Autodesk Inventor part; units mm, degrees
(part 3 of 5)
  line L98 (0, 22) -> (0, -22) construction
  circle A131 centre (-90.3659, 45.1111) radius 1.6
  circle A132 centre (-45.1111, 90.3659) radius 1.6
  circle A133 centre (90.3659, -45.1111) radius 1.6
  circle A134 centre (45.1111, -90.3659) radius 1.6
  circle A135 centre (90.3659, 45.1111) radius 1.6
  circle A136 centre (45.1111, 90.3659) radius 1.6
  line L99 (41.3657, 27.2236) -> (27.2236, 41.3657) construction
  line L100 (34.2947, 34.2947) -> (55.1543, 55.1543) construction
  line L101 (46.669, 63.6396) -> (63.6396, 46.669) construction
  line L102 (0, 0) -> (0, -61.2072) construction
  circle A137 centre (0, -54) radius 1.6
  arc A138 (3.4868, -52.0398) -> (-3.4868, -52.0398) centre (0, -54) ccw
  line L103 (-0.6161, -51.9466) -> (-14.5119, -56.4463) construction
  line L104 (-5.1776, -53.4237) -> (-14.5119, -56.4463) construction
  line L105 (14.5119, -56.4463) -> (0.6161, -51.9466) construction
  line L106 (5.1776, -53.4237) -> (14.5119, -56.4463) construction
  arc A139 (0, -58) -> (3.8733, -53.0013) centre (0, -54) ccw construction
  arc A140 (-3.8733, -53.0013) -> (0, -58) centre (0, -54) ccw construction
  arc A141 (-5.1776, -53.4237) -> (-3.4868, -52.0398) centre (-6.1018, -50.5696) ccw
  arc A142 (3.4868, -52.0398) -> (5.1776, -53.4237) centre (6.1018, -50.5696) ccw
  line L107 (5.1776, -53.4237) -> (3.794, -57.2809)
  line L108 (3.794, -57.2809) -> (-2.6441, -58)
  line L109 (-2.6441, -58) -> (-5.1776, -53.4237)
  dimension "d114" = 3.2
  dimension "d117" = 64
  dimension "d118" = 3.2
  dimension "d119" = 54
  dimension "d120" = 8
  dimension "d121" = 3
  constraints: 20 end point, 15 centre point, 14 point on circle, 7 symmetric about line, 6 point on line, 4 midpoint, 4 tangent, 2 coincident, 2 collinear, 2 vertical, 1 equal radius, 1 horizontal, 7 other
  measures "d114" diameter of A129
  measures "d117" distance of A135.centre A136.centre
  measures "d118" diameter of A137
  measures "d119" distance of A137.centre point (0, 0)
  measures "d120" diameter of A138
  measures "d121" radius of A141
extrude "Выдавливание9" cut sketch "Эскиз6" against normal blind 10 contours A129 | A130 | A131 | A132 | A133 | A134 | A135 | A136 | A137
extrude "Выдавливание10" add sketch "Эскиз6" against normal blind 2 contours A142 L107 L108 L109 A141 A138
sketch "Эскиз7" plane through (0, 2, 0) normal (0, 1, 0) x (1, 0, 0)
  line L0 (-25, -33.1335) -> (25, -33.1335) construction
  line L1 (25, -33.1335) -> (25, -43.1335) construction
  line L2 (25, -43.1335) -> (-25, -43.1335) construction
  line L3 (-25, -43.1335) -> (-25, -33.1335) construction
  line L4 (0, 0) -> (0, -69.4501) construction
  circle A0 centre (21.9203, -43.1335) radius 1.6 construction
  circle A1 centre (-21.9203, -43.1335) radius 1.6 construction
  dimension "d124" = 50
  dimension "d125" = 10
  constraints: 10 end point, 2 parallel, 1 horizontal, 1 perpendicular, 1 point on line, 1 vertical, 1 other
  measures "d124" distance of L1.end L2.end
  measures "d125" distance of L0.end L1.end
sketch "Эскиз8" plane through (0, 0, 0) normal (0, -1, 0) x (1, 0, 0)
  circle A0 centre (0, 54) radius 1.6 construction
  line L0 (14.5119, 56.4463) -> (5.1776, 53.4237) construction
  arc A1 (15.1585, 56.5907) -> (14.5119, 56.4463) centre (15.6055, 53.069) ccw construction
  line L1 (20.596, 57.2809) -> (15.1585, 56.5907) construction
  line L2 (20.596, 57.2809) -> (26.2105, 51.6664) construction
  line L3 (26.2105, 51.6664) -> (21.6698, 47.1257) construction
  arc A2 (21.6698, 47.1257) -> (17.9282, 43.384) centre (21.9203, 43.1335) ccw construction
  line L4 (17.9282, 43.384) -> (1.4142, 26.8701) construction
  arc A3 (-1.4142, 26.8701) -> (1.4142, 26.8701) centre (0, 28.2843) ccw construction
  line L5 (-1.4142, 26.8701) -> (-17.9282, 43.384) construction
  arc A4 (-17.9282, 43.384) -> (-21.6698, 47.1257) centre (-21.9203, 43.1335) ccw construction
  line L6 (-21.6698, 47.1257) -> (-26.2105, 51.6664) construction
  line L7 (-26.2105, 51.6664) -> (-20.596, 57.2809) construction
  line L8 (-15.1585, 56.5907) -> (-20.596, 57.2809) construction
  arc A5 (-14.5119, 56.4463) -> (-15.1585, 56.5907) centre (-15.6055, 53.069) ccw construction
  line L9 (-5.1776, 53.4237) -> (-14.5119, 56.4463) construction
  arc A6 (-3.4868, 52.0398) -> (-5.1776, 53.4237) centre (-6.1018, 50.5696) ccw construction
  arc A7 (-3.4868, 52.0398) -> (3.4868, 52.0398) centre (0, 54) ccw construction
  arc A8 (5.1776, 53.4237) -> (3.4868, 52.0398) centre (6.1018, 50.5696) ccw construction
  circle A9 centre (45.1111, 90.3659) radius 1.6 construction
  circle A10 centre (-45.1111, -90.3659) radius 1.6 construction
  circle A11 centre (-90.3659, -45.1111) radius 1.6 construction
  circle A12 centre (90.3659, 45.1111) radius 1.6 construction
  circle A13 centre (-45.1111, 90.3659) radius 1.6 construction
  circle A14 centre (45.1111, -90.3659) radius 1.6 construction
  circle A15 centre (-90.3659, 45.1111) radius 1.6 construction
  circle A16 centre (90.3659, -45.1111) radius 1.6 construction
  circle A17 centre (101, 0) radius 1.6 construction
  circle A18 centre (-101, 0) radius 1.6 construction
  arc A19 (-93.0503, 48.6481) -> (-93.0503, -48.6481) centre (0, 0) ccw construction
  arc A20 (-93.0503, -48.6481) -> (-88.2704, -49.3795) centre (-90.3917, -47.2582) ccw construction
  line L10 (-85.2064, -46.3155) -> (-88.2704, -49.3795) construction
  arc A21 (-73.8927, -46.3155) -> (-85.2064, -46.3155) centre (-79.5495, -51.9723) ccw construction
  line L11 (-46.3155, -73.8927) -> (-73.8927, -46.3155) construction
  arc A22 (-46.3155, -85.2064) -> (-46.3155, -73.8927) centre (-51.9723, -79.5495) ccw construction
  line L12 (-49.3795, -88.2704) -> (-46.3155, -85.2064) construction
  arc A23 (-49.3795, -88.2704) -> (-48.6481, -93.0503) centre (-47.2582, -90.3917) ccw construction
  arc A24 (-48.6481, -93.0503) -> (-11.8382, -104.3305) centre (0, 0) ccw construction
  arc A25 (-11.8382, -104.3305) -> (-8.5, -101.3496) centre (-11.5, -101.3496) ccw construction
  line L13 (-8.5, -101.3496) -> (-8.5, -90.5) construction
  arc A26 (-7, -89) -> (-8.5, -90.5) centre (-7, -90.5) ccw construction
  line L14 (-7, -89) -> (7, -89) construction
  arc A27 (8.5, -90.5) -> (7, -89) centre (7, -90.5) ccw construction
  line L15 (8.5, -90.5) -> (8.5, -101.3496) construction
  arc A28 (8.5, -101.3496) -> (11.8382, -104.3305) centre (11.5, -101.3496) ccw construction
  arc A29 (11.8382, -104.3305) -> (48.6481, -93.0503) centre (0, 0) ccw construction
  arc A30 (48.6481, -93.0503) -> (49.3795, -88.2704) centre (47.2582, -90.3917) ccw construction
  line L16 (46.3155, -85.2064) -> (49.3795, -88.2704) construction
  arc A31 (46.3155, -73.8927) -> (46.3155, -85.2064) centre (51.9723, -79.5495) ccw construction
  line L17 (73.8927, -46.3155) -> (46.3155, -73.8927) construction
  arc A32 (85.2064, -46.3155) -> (73.8927, -46.3155) centre (79.5495, -51.9723) ccw construction
  line L18 (88.2704, -49.3795) -> (85.2064, -46.3155) construction
  arc A33 (88.2704, -49.3795) -> (93.0503, -48.6481) centre (90.3917, -47.2582) ccw construction
  arc A34 (93.0503, -48.6481) -> (93.0503, 48.6481) centre (0, 0) ccw construction
  arc A35 (93.0503, 48.6481) -> (88.2704, 49.3795) centre (90.3917, 47.2582) ccw construction
  line L19 (85.2064, 46.3155) -> (88.2704, 49.3795) construction
  arc A36 (73.8927, 46.3155) -> (85.2064, 46.3155) centre (79.5495, 51.9723) ccw construction
  line L20 (46.3155, 73.8927) -> (73.8927, 46.3155) construction
  arc A37 (46.3155, 85.2064) -> (46.3155, 73.8927) centre (51.9723, 79.5495) ccw construction
  line L21 (49.3795, 88.2704) -> (46.3155, 85.2064) construction
  arc A38 (49.3795, 88.2704) -> (48.6481, 93.0503) centre (47.2582, 90.3917) ccw construction
  arc A39 (48.6481, 93.0503) -> (45.42, 94.668) centre (0, 0) ccw construction
  arc A40 (45.42, 94.668) -> (43.0355, 94.1655) centre (44.5548, 92.8648) ccw construction
  line L22 (18.3802, 65.3664) -> (43.0355, 94.1655) construction
  arc A41 (17.477, 64.7643) -> (18.3802, 65.3664) centre (16.8609, 66.6671) ccw construction
  line L23 (0.6161, 59.3045) -> (17.477, 64.7643) construction
  arc A42 (-0.6161, 59.3045) -> (0.6161, 59.3045) centre (0, 61.2072) ccw construction
  line L24 (-17.477, 64.7643) -> (-0.6161, 59.3045) construction
  arc A43 (-18.3802, 65.3664) -> (-17.477, 64.7643) centre (-16.8609, 66.6671) ccw construction
  line L25 (-43.0355, 94.1655) -> (-18.3802, 65.3664) construction
  arc A44 (-43.0355, 94.1655) -> (-45.42, 94.668) centre (-44.5548, 92.8648) ccw construction
  arc A45 (-45.42, 94.668) -> (-48.6481, 93.0503) centre (0, 0) ccw construction
  arc A46 (-48.6481, 93.0503) -> (-49.3795, 88.2704) centre (-47.2582, 90.3917) ccw construction
  line L26 (-46.3155, 85.2064) -> (-49.3795, 88.2704) construction
  arc A47 (-46.3155, 73.8927) -> (-46.3155, 85.2064) centre (-51.9723, 79.5495) ccw construction
  line L27 (-73.8927, 46.3155) -> (-46.3155, 73.8927) construction
  arc A48 (-85.2064, 46.3155) -> (-73.8927, 46.3155) centre (-79.5495, 51.9723) ccw construction
  line L28 (-88.2704, 49.3795) -> (-85.2064, 46.3155) construction
  arc A49 (-88.2704, 49.3795) -> (-93.0503, 48.6481) centre (-90.3917, 47.2582) ccw construction
  arc A50 (90.4395, -37.7453) -> (97.9653, -2.6059) centre (0, 0) ccw construction
  arc A51 (87.1795, -38.3892) -> (90.4395, -37.7453) centre (88.5938, -36.975) ccw construction
  line L29 (83.085, -34.2947) -> (87.1795, -38.3892) construction
  arc A52 (83.085, -34.2947) -> (76.014, -34.2947) centre (79.5495, -37.8302) ccw construction
  line L30 (67.8823, -42.4264) -> (76.014, -34.2947) construction
  line L31 (67.8823, -42.4264) -> (47.1257, -21.6698) construction
  arc A53 (47.1257, -21.6698) -> (43.384, -17.9282) centre (43.1335, -21.9203) ccw construction
  line L32 (43.384, -17.9282) -> (26.8701, -1.4142) construction
  arc A54 (26.8701, 1.4142) -> (26.8701, -1.4142) centre (28.2843, 0) ccw construction
  line L33 (26.8701, 1.4142) -> (43.384, 17.9282) construction
  arc A55 (43.384, 17.9282) -> (47.1257, 21.6698) centre (43.1335, 21.9203) ccw construction
  line L34 (47.1257, 21.6698) -> (67.8823, 42.4264) construction
  line L35 (76.014, 34.2947) -> (67.8823, 42.4264) construction
  arc A56 (76.014, 34.2947) -> (83.085, 34.2947) centre (79.5495, 37.8302) ccw construction
  line L36 (87.1795, 38.3892) -> (83.085, 34.2947) construction
  arc A57 (90.4395, 37.7453) -> (87.1795, 38.3892) centre (88.5938, 36.975) ccw construction
  arc A58 (97.9653, 2.6059) -> (90.4395, 37.7453) centre (0, 0) ccw construction
  arc A59 (97.9653, 2.6059) -> (97.9653, -2.6059) centre (101, 0) ccw construction
  line L37 (29.746, 55.2019) -> (24.3148, 60.6331) construction
  line L38 (24.842, 61.8893) -> (24.3148, 60.6331) construction
  arc A60 (25.4187, 62.8242) -> (24.842, 61.8893) centre (28.1154, 60.5155) ccw construction
  line L39 (34.1909, 73.0707) -> (25.4187, 62.8242) construction
  arc A61 (37.1244, 73.1843) -> (34.1909, 73.0707) centre (35.7102, 71.7701) ccw construction
  line L40 (42.4264, 67.8823) -> (37.1244, 73.1843) construction
  line L41 (42.4264, 67.8823) -> (29.746, 55.2019) construction
  arc A62 (14.5, -93.3742) -> (18.0526, -96.3229) centre (17.5, -93.3742) ccw construction
  line L42 (14.5, -93.3742) -> (14.5, -87) construction
  arc A63 (14.5, -87) -> (11.5, -84) centre (11.5, -87) ccw construction
  line L43 (11.5, -84) -> (-11.5, -84) construction
  arc A64 (-11.5, -84) -> (-14.5, -87) centre (-11.5, -87) ccw construction
  line L44 (-14.5, -87) -> (-14.5, -93.3742) construction
  arc A65 (-18.0526, -96.3229) -> (-14.5, -93.3742) centre (-17.5, -93.3742) ccw construction
  arc A66 (-37.7453, -90.4395) -> (-18.0526, -96.3229) centre (0, 0) ccw construction
  arc A67 (-38.3892, -87.1795) -> (-37.7453, -90.4395) centre (-36.975, -88.5938) ccw construction
  line L45 (-34.2947, -83.085) -> (-38.3892, -87.1795) construction
  arc A68 (-34.2947, -83.085) -> (-34.2947, -76.014) centre (-37.8302, -79.5495) ccw construction
  line L46 (-42.4264, -67.8823) -> (-34.2947, -76.014) construction
  line L47 (-42.4264, -67.8823) -> (-21.6698, -47.1257) construction
  arc A69 (-21.6698, -47.1257) -> (-17.9282, -43.384) centre (-21.9203, -43.1335) ccw construction
  line L48 (-17.9282, -43.384) -> (-1.4142, -26.8701) construction
  arc A70 (1.4142, -26.8701) -> (-1.4142, -26.8701) centre (0, -28.2843) ccw construction
  line L49 (1.4142, -26.8701) -> (17.9282, -43.384) construction
  arc A71 (17.9282, -43.384) -> (21.6698, -47.1257) centre (21.9203, -43.1335) ccw construction
  line L50 (21.6698, -47.1257) -> (42.4264, -67.8823) construction
  line L51 (34.2947, -76.014) -> (42.4264, -67.8823) construction
  arc A72 (34.2947, -76.014) -> (34.2947, -83.085) centre (37.8302, -79.5495) ccw construction
  line L52 (38.3892, -87.1795) -> (34.2947, -83.085) construction
  arc A73 (37.7453, -90.4395) -> (38.3892, -87.1795) centre (36.975, -88.5938) ccw construction
  arc A74 (18.0526, -96.3229) -> (37.7453, -90.4395) centre (0, 0) ccw construction
  line L53 (63.6396, 46.669) -> (46.669, 63.6396) construction
  line L54 (63.6396, 46.669) -> (44.1942, 27.2236) construction
  arc A75 (41.3657, 27.2236) -> (44.1942, 27.2236) centre (42.78, 28.6378) ccw construction
  line L55 (41.3657, 27.2236) -> (27.2236, 41.3657) construction
  arc A76 (27.2236, 44.1942) -> (27.2236, 41.3657) centre (28.6378, 42.78) ccw construction
  line L56 (27.2236, 44.1942) -> (46.669, 63.6396) construction
  line L57 (46.669, -63.6396) -> (63.6396, -46.669) construction
  line L58 (46.669, -63.6396) -> (27.2236, -44.1942) construction
  arc A77 (27.2236, -41.3657) -> (27.2236, -44.1942) centre (28.6378, -42.78) ccw construction
  line L59 (27.2236, -41.3657) -> (41.3657, -27.2236) construction
  arc A78 (44.1942, -27.2236) -> (41.3657, -27.2236) centre (42.78, -28.6378) ccw construction
  line L60 (44.1942, -27.2236) -> (63.6396, -46.669) construction
  line L61 (-63.6396, -46.669) -> (-46.669, -63.6396) construction
  line L62 (-63.6396, -46.669) -> (-44.1942, -27.2236) construction
  arc A79 (-41.3657, -27.2236) -> (-44.1942, -27.2236) centre (-42.78, -28.6378) ccw construction
  line L63 (-41.3657, -27.2236) -> (-27.2236, -41.3657) construction
  arc A80 (-27.2236, -44.1942) -> (-27.2236, -41.3657) centre (-28.6378, -42.78) ccw construction
  line L64 (-27.2236, -44.1942) -> (-46.669, -63.6396) construction
  line L65 (-46.669, 63.6396) -> (-63.6396, 46.669) construction
  line L66 (-46.669, 63.6396) -> (-27.2236, 44.1942) construction
  arc A81 (-27.2236, 41.3657) -> (-27.2236, 44.1942) centre (-28.6378, 42.78) ccw construction
  line L67 (-27.2236, 41.3657) -> (-41.3657, 27.2236) construction
  arc A82 (-44.1942, 27.2236) -> (-41.3657, 27.2236) centre (-42.78, 28.6378) ccw construction
  line L68 (-44.1942, 27.2236) -> (-63.6396, 46.669) construction
  arc A83 (7.7166, 24.6871) -> (8.4003, 21.4111) centre (9.1308, 23.2729) ccw construction
  line L69 (7.7166, 24.6871) -> (20.8597, 37.8302) construction
  arc A84 (23.6881, 37.8302) -> (20.8597, 37.8302) centre (22.2739, 36.416) ccw construction
  line L70 (23.6881, 37.8302) -> (37.8302, 23.6881) construction
  arc A85 (37.8302, 20.8597) -> (37.8302, 23.6881) centre (36.416, 22.2739) ccw construction
  line L71 (37.8302, 20.8597) -> (24.6871, 7.7166) construction
  arc A86 (21.4111, 8.4003) -> (24.6871, 7.7166) centre (23.2729, 9.1308) ccw construction
  arc A87 (21.4111, 8.4003) -> (8.4003, 21.4111) centre (0, 0) ccw construction
  circle A88 centre (-21.9203, -43.1335) radius 1.6 construction
  arc A89 (-21.4111, -8.4003) -> (-24.6871, -7.7166) centre (-23.2729, -9.1308) ccw construction
  arc A90 (-21.4111, -8.4003) -> (-8.4003, -21.4111) centre (0, 0) ccw construction
  arc A91 (-7.7166, -24.6871) -> (-8.4003, -21.4111) centre (-9.1308, -23.2729) ccw construction
  line L72 (-7.7166, -24.6871) -> (-20.8597, -37.8302) construction
  arc A92 (-23.6881, -37.8302) -> (-20.8597, -37.8302) centre (-22.2739, -36.416) ccw construction
  line L73 (-23.6881, -37.8302) -> (-37.8302, -23.6881) construction
  arc A93 (-37.8302, -20.8597) -> (-37.8302, -23.6881) centre (-36.416, -22.2739) ccw construction
  line L74 (-37.8302, -20.8597) -> (-24.6871, -7.7166) construction
  line L75 (24.6871, -7.7166) -> (37.8302, -20.8597) construction
  arc A94 (37.8302, -23.6881) -> (37.8302, -20.8597) centre (36.416, -22.2739) ccw construction
  line L76 (37.8302, -23.6881) -> (23.6881, -37.8302) construction
  arc A95 (20.8597, -37.8302) -> (23.6881, -37.8302) centre (22.2739, -36.416) ccw construction
  line L77 (20.8597, -37.8302) -> (7.7166, -24.6871) construction
  arc A96 (8.4003, -21.4111) -> (7.7166, -24.6871) centre (9.1308, -23.2729) ccw construction
  arc A97 (8.4003, -21.4111) -> (21.4111, -8.4003) centre (0, 0) ccw construction
  arc A98 (24.6871, -7.7166) -> (21.4111, -8.4003) centre (23.2729, -9.1308) ccw construction
  circle A99 centre (21.9203, 43.1335) radius 1.6 construction
  line L78 (-37.8302, 23.6881) -> (-23.6881, 37.8302) construction
  arc A100 (-20.8597, 37.8302) -> (-23.6881, 37.8302) centre (-22.2739, 36.416) ccw construction
  line L79 (-20.8597, 37.8302) -> (-7.7166, 24.6871) construction
  arc A101 (-8.4003, 21.4111) -> (-7.7166, 24.6871) centre (-9.1308, 23.2729) ccw construction
  arc A102 (-8.4003, 21.4111) -> (-21.4111, 8.4003) centre (0, 0) ccw construction
  arc A103 (-24.6871, 7.7166) -> (-21.4111, 8.4003) centre (-23.2729, 9.1308) ccw construction
  line L80 (-24.6871, 7.7166) -> (-37.8302, 20.8597) construction
  arc A104 (-37.8302, 23.6881) -> (-37.8302, 20.8597) centre (-36.416, 22.2739) ccw construction
  circle A105 centre (-43.1335, 21.9203) radius 1.6 construction
  circle A106 centre (43.1335, -21.9203) radius 1.6 construction
  circle A107 centre (21.9203, -43.1335) radius 1.6 construction
  circle A108 centre (-21.9203, 43.1335) radius 1.6 construction
  circle A109 centre (-43.1335, -21.9203) radius 1.6 construction
  circle A110 centre (0, 0) radius 18 construction
  circle A111 centre (43.1335, 21.9203) radius 1.6 construction
  circle A112 centre (0, -22) radius 1.6 construction
  circle A113 centre (-22, 0) radius 1.6 construction
  circle A114 centre (0, 22) radius 1.6 construction
  circle A115 centre (22, 0) radius 1.6 construction
  circle A116 centre (-37.8302, -79.5495) radius 1.6 construction
  circle A117 centre (-79.5495, -37.8302) radius 1.6 construction
  circle A118 centre (-79.5495, 37.8302) radius 1.6 construction
  circle A119 centre (79.5495, 37.8302) radius 1.6 construction
  circle A120 centre (37.8302, -79.5495) radius 1.6 construction
  circle A121 centre (79.5495, -37.8302) radius 1.6 construction
  circle A122 centre (-20.5578, 60.8546) radius 1.55 construction
  circle A123 centre (20.5578, 60.8546) radius 1.55 construction
  circle A124 centre (37.8302, 79.5495) radius 1.6 construction
  circle A125 centre (-37.8302, 79.5495) radius 1.6 construction
  line L81 (-24.3148, 60.6331) -> (-29.746, 55.2019) construction
  line L82 (-29.746, 55.2019) -> (-42.4264, 67.8823) construction
  line L83 (-37.1244, 73.1843) -> (-42.4264, 67.8823) construction
  arc A126 (-34.1909, 73.0707) -> (-37.1244, 73.1843) centre (-35.7102, 71.7701) ccw construction
  line L84 (-25.4187, 62.8242) -> (-34.1909, 73.0707) construction
  arc A127 (-24.842, 61.8893) -> (-25.4187, 62.8242) centre (-28.1154, 60.5155) ccw construction
  line L85 (-24.3148, 60.6331) -> (-24.842, 61.8893) construction
  arc A128 (-90.4395, 37.7453) -> (-97.9653, 2.6059) centre (0, 0) ccw construction
  arc A129 (-87.1795, 38.3892) -> (-90.4395, 37.7453) centre (-88.5938, 36.975) ccw construction
  line L86 (-83.085, 34.2947) -> (-87.1795, 38.3892) construction
  arc A130 (-83.085, 34.2947) -> (-76.014, 34.2947) centre (-79.5495, 37.8302) ccw construction
  line L87 (-67.8823, 42.4264) -> (-76.014, 34.2947) construction
  line L88 (-67.8823, 42.4264) -> (-47.1257, 21.6698) construction
  arc A131 (-47.1257, 21.6698) -> (-43.384, 17.9282) centre (-43.1335, 21.9203) ccw construction
  line L89 (-43.384, 17.9282) -> (-26.8701, 1.4142) construction
  arc A132 (-26.8701, -1.4142) -> (-26.8701, 1.4142) centre (-28.2843, 0) ccw construction
  line L90 (-26.8701, -1.4142) -> (-43.384, -17.9282) construction
  arc A133 (-43.384, -17.9282) -> (-47.1257, -21.6698) centre (-43.1335, -21.9203) ccw construction
  line L91 (-47.1257, -21.6698) -> (-67.8823, -42.4264) construction
  line L92 (-76.014, -34.2947) -> (-67.8823, -42.4264) construction
  arc A134 (-76.014, -34.2947) -> (-83.085, -34.2947) centre (-79.5495, -37.8302) ccw construction
  line L93 (-87.1795, -38.3892) -> (-83.085, -34.2947) construction
  arc A135 (-90.4395, -37.7453) -> (-87.1795, -38.3892) centre (-88.5938, -36.975) ccw construction
  arc A136 (-97.9653, -2.6059) -> (-90.4395, -37.7453) centre (0, 0) ccw construction
  arc A137 (-97.9653, -2.6059) -> (-97.9653, 2.6059) centre (-101, 0) ccw construction
  line L94 (19.5177, 122.3748) -> (96.2153, 45.6773) construction
  arc A138 (93.0503, 48.6481) -> (88.2704, 49.3795) centre (90.3917, 47.2582) ccw construction
  line L95 (-105.344, -36.5485) -> (-36.5776, -105.315) construction
  arc A139 (-49.3795, -88.2704) -> (-48.6481, -93.0503) centre (-47.2582, -90.3917) ccw construction
  arc A140 (-93.0503, -48.6481) -> (-88.2704, -49.3795) centre (-90.3917, -47.2582) ccw construction
  dimension "d126" = 200.6664
  constraints: 4 end point, 4 tangent
  measures "d126" distance between parallel lines of L94 L95
sketch "Эскиз9" plane through (0, 2, 0) normal (0, 1, 0) x (1, 0, 0)
  circle A0 centre (-21.9203, -33.1335) radius 1.6
  line L0 (0, -22.0571) -> (0, -53.9754) construction
  circle A1 centre (0, -54) radius 1.6 construction
  arc A2 (-93.0503, 48.6481) -> (-93.0503, -48.6481) centre (0, 0) ccw construction
  arc A3 (-93.0503, -48.6481) -> (-88.2704, -49.3795) centre (-90.3917, -47.2582) ccw construction
  line L1 (-88.2704, -49.3795) -> (-85.2064, -46.3155) construction
  arc A4 (-73.8927, -46.3155) -> (-85.2064, -46.3155) centre (-79.5495, -51.9723) ccw construction
  line L2 (-73.8927, -46.3155) -> (-46.3155, -73.8927) construction
  arc A5 (-46.3155, -85.2064) -> (-46.3155, -73.8927) centre (-51.9723, -79.5495) ccw construction
  line L3 (-46.3155, -85.2064) -> (-49.3795, -88.2704) construction
  arc A6 (-49.3795, -88.2704) -> (-48.6481, -93.0503) centre (-47.2582, -90.3917) ccw construction
  arc A7 (-48.6481, -93.0503) -> (-45.42, -94.668) centre (0, 0) ccw construction
  arc A8 (-45.42, -94.668) -> (-43.0355, -94.1655) centre (-44.5548, -92.8648) ccw construction
  line L4 (-43.0355, -94.1655) -> (-18.3802, -65.3664) construction
  arc A9 (-17.477, -64.7643) -> (-18.3802, -65.3664) centre (-16.8609, -66.6671) ccw construction
  line L5 (-17.477, -64.7643) -> (-0.6161, -59.3045) construction
  arc A10 (0.6161, -59.3045) -> (-0.6161, -59.3045) centre (0, -61.2072) ccw construction
  line L6 (0.6161, -59.3045) -> (17.477, -64.7643) construction
  arc A11 (18.3802, -65.3664) -> (17.477, -64.7643) centre (16.8609, -66.6671) ccw construction
  line L7 (18.3802, -65.3664) -> (43.0355, -94.1655) construction
  arc A12 (43.0355, -94.1655) -> (45.42, -94.668) centre (44.5548, -92.8648) ccw construction
  arc A13 (45.42, -94.668) -> (48.6481, -93.0503) centre (0, 0) ccw construction
  arc A14 (48.6481, -93.0503) -> (49.3795, -88.2704) centre (47.2582, -90.3917) ccw construction
  line L8 (49.3795, -88.2704) -> (46.3155, -85.2064) construction
  arc A15 (46.3155, -73.8927) -> (46.3155, -85.2064) centre (51.9723, -79.5495) ccw construction
  line L9 (46.3155, -73.8927) -> (73.8927, -46.3155) construction
  arc A16 (85.2064, -46.3155) -> (73.8927, -46.3155) centre (79.5495, -51.9723) ccw construction
  line L10 (85.2064, -46.3155) -> (88.2704, -49.3795) construction
  arc A17 (88.2704, -49.3795) -> (93.0503, -48.6481) centre (90.3917, -47.2582) ccw construction
  arc A18 (93.0503, -48.6481) -> (93.0503, 48.6481) centre (0, 0) ccw construction
  arc A19 (93.0503, 48.6481) -> (88.2704, 49.3795) centre (90.3917, 47.2582) ccw construction
  line L11 (88.2704, 49.3795) -> (85.2064, 46.3155) construction
  arc A20 (73.8927, 46.3155) -> (85.2064, 46.3155) centre (79.5495, 51.9723) ccw construction
  line L12 (73.8927, 46.3155) -> (46.3155, 73.8927) construction
  arc A21 (46.3155, 85.2064) -> (46.3155, 73.8927) centre (51.9723, 79.5495) ccw construction
  line L13 (46.3155, 85.2064) -> (49.3795, 88.2704) construction
  arc A22 (49.3795, 88.2704) -> (48.6481, 93.0503) centre (47.2582, 90.3917) ccw construction
  arc A23 (48.6481, 93.0503) -> (11.8382, 104.3305) centre (0, 0) ccw construction
  arc A24 (11.8382, 104.3305) -> (8.5, 101.3496) centre (11.5, 101.3496) ccw construction
  line L14 (8.5, 101.3496) -> (8.5, 90.5) construction
  arc A25 (7, 89) -> (8.5, 90.5) centre (7, 90.5) ccw construction
  line L15 (7, 89) -> (-7, 89) construction
  arc A26 (-8.5, 90.5) -> (-7, 89) centre (-7, 90.5) ccw construction
  line L16 (-8.5, 90.5) -> (-8.5, 101.3496) construction
  arc A27 (-8.5, 101.3496) -> (-11.8382, 104.3305) centre (-11.5, 101.3496) ccw construction
  arc A28 (-11.8382, 104.3305) -> (-48.6481, 93.0503) centre (0, 0) ccw construction
  arc A29 (-48.6481, 93.0503) -> (-49.3795, 88.2704) centre (-47.2582, 90.3917) ccw construction
  line L17 (-49.3795, 88.2704) -> (-46.3155, 85.2064) construction
  arc A30 (-46.3155, 73.8927) -> (-46.3155, 85.2064) centre (-51.9723, 79.5495) ccw construction
  line L18 (-46.3155, 73.8927) -> (-73.8927, 46.3155) construction
  arc A31 (-85.2064, 46.3155) -> (-73.8927, 46.3155) centre (-79.5495, 51.9723) ccw construction
  line L19 (-85.2064, 46.3155) -> (-88.2704, 49.3795) construction
  arc A32 (-88.2704, 49.3795) -> (-93.0503, 48.6481) centre (-90.3917, 47.2582) ccw construction
  arc A33 (-90.4395, 37.7453) -> (-97.9653, 2.6059) centre (0, 0) ccw construction
  arc A34 (-87.1795, 38.3892) -> (-90.4395, 37.7453) centre (-88.5938, 36.975) ccw construction
  line L20 (-87.1795, 38.3892) -> (-83.085, 34.2947) construction
  arc A35 (-83.085, 34.2947) -> (-76.014, 34.2947) centre (-79.5495, 37.8302) ccw construction
  line L21 (-76.014, 34.2947) -> (-67.8823, 42.4264) construction
  line L22 (-67.8823, 42.4264) -> (-47.1257, 21.6698) construction
  arc A36 (-47.1257, 21.6698) -> (-43.384, 17.9282) centre (-43.1335, 21.9203) ccw construction
  line L23 (-43.384, 17.9282) -> (-26.8701, 1.4142) construction
  arc A37 (-26.8701, -1.4142) -> (-26.8701, 1.4142) centre (-28.2843, 0) ccw construction
  line L24 (-26.8701, -1.4142) -> (-43.384, -17.9282) construction
  arc A38 (-43.384, -17.9282) -> (-47.1257, -21.6698) centre (-43.1335, -21.9203) ccw construction
  line L25 (-47.1257, -21.6698) -> (-67.8823, -42.4264) construction
  line L26 (-67.8823, -42.4264) -> (-76.014, -34.2947) construction
  arc A39 (-76.014, -34.2947) -> (-83.085, -34.2947) centre (-79.5495, -37.8302) ccw construction
  line L27 (-83.085, -34.2947) -> (-87.1795, -38.3892) construction
  arc A40 (-90.4395, -37.7453) -> (-87.1795, -38.3892) centre (-88.5938, -36.975) ccw construction
  arc A41 (-97.9653, -2.6059) -> (-90.4395, -37.7453) centre (0, 0) ccw construction
  arc A42 (-97.9653, -2.6059) -> (-97.9653, 2.6059) centre (-101, 0) ccw construction
  line L28 (29.746, -55.2019) -> (42.4264, -67.8823) construction
  line L29 (42.4264, -67.8823) -> (37.1244, -73.1843) construction
  arc A43 (34.1909, -73.0707) -> (37.1244, -73.1843) centre (35.7102, -71.7701) ccw construction
  line L30 (34.1909, -73.0707) -> (25.4187, -62.8242) construction
  arc A44 (24.842, -61.8893) -> (25.4187, -62.8242) centre (28.1154, -60.5155) ccw construction
  line L31 (24.842, -61.8893) -> (24.3148, -60.6331) construction
  line L32 (24.3148, -60.6331) -> (29.746, -55.2019) construction
  line L33 (-24.3148, -60.6331) -> (-24.842, -61.8893) construction
  arc A45 (-25.4187, -62.8242) -> (-24.842, -61.8893) centre (-28.1154, -60.5155) ccw construction
  line L34 (-25.4187, -62.8242) -> (-34.1909, -73.0707) construction
  arc A46 (-37.1244, -73.1843) -> (-34.1909, -73.0707) centre (-35.7102, -71.7701) ccw construction
  line L35 (-37.1244, -73.1843) -> (-42.4264, -67.8823) construction
  line L36 (-42.4264, -67.8823) -> (-29.746, -55.2019) construction
  line L37 (-29.746, -55.2019) -> (-24.3148, -60.6331) construction
  arc A47 (37.7453, 90.4395) -> (18.0526, 96.3229) centre (0, 0) ccw construction
  arc A48 (38.3892, 87.1795) -> (37.7453, 90.4395) centre (36.975, 88.5938) ccw construction
  line L38 (38.3892, 87.1795) -> (34.2947, 83.085) construction
  arc A49 (34.2947, 83.085) -> (34.2947, 76.014) centre (37.8302, 79.5495) ccw construction
  line L39 (34.2947, 76.014) -> (42.4264, 67.8823) construction
  line L40 (42.4264, 67.8823) -> (21.6698, 47.1257) construction
  arc A50 (21.6698, 47.1257) -> (17.9282, 43.384) centre (21.9203, 43.1335) ccw construction
  line L41 (17.9282, 43.384) -> (1.4142, 26.8701) construction
  arc A51 (-1.4142, 26.8701) -> (1.4142, 26.8701) centre (0, 28.2843) ccw construction
  line L42 (-1.4142, 26.8701) -> (-17.9282, 43.384) construction
  arc A52 (-17.9282, 43.384) -> (-21.6698, 47.1257) centre (-21.9203, 43.1335) ccw construction
  line L43 (-21.6698, 47.1257) -> (-42.4264, 67.8823) construction
  line L44 (-42.4264, 67.8823) -> (-34.2947, 76.014) construction
  arc A53 (-34.2947, 76.014) -> (-34.2947, 83.085) centre (-37.8302, 79.5495) ccw construction
  line L45 (-34.2947, 83.085) -> (-38.3892, 87.1795) construction
  arc A54 (-37.7453, 90.4395) -> (-38.3892, 87.1795) centre (-36.975, 88.5938) ccw construction
  arc A55 (-18.0526, 96.3229) -> (-37.7453, 90.4395) centre (0, 0) ccw construction
  arc A56 (-14.5, 93.3742) -> (-18.0526, 96.3229) centre (-17.5, 93.3742) ccw construction
  line L46 (-14.5, 93.3742) -> (-14.5, 87) construction
  arc A57 (-14.5, 87) -> (-11.5, 84) centre (-11.5, 87) ccw construction
  line L47 (-11.5, 84) -> (11.5, 84) construction
  arc A58 (11.5, 84) -> (14.5, 87) centre (11.5, 87) ccw construction
  line L48 (14.5, 87) -> (14.5, 93.3742) construction
  arc A59 (18.0526, 96.3229) -> (14.5, 93.3742) centre (17.5, 93.3742) ccw construction
  line L49 (-63.6396, -46.669) -> (-44.1942, -27.2236) construction
  arc A60 (-41.3657, -27.2236) -> (-44.1942, -27.2236) centre (-42.78, -28.6378) ccw construction
  line L50 (-41.3657, -27.2236) -> (-27.2236, -41.3657) construction
  arc A61 (-27.2236, -44.1942) -> (-27.2236, -41.3657) centre (-28.6378, -42.78) ccw construction
  line L51 (-27.2236, -44.1942) -> (-46.669, -63.6396) construction
  line L52 (-46.669, -63.6396) -> (-63.6396, -46.669) construction
  circle A62 centre (-37.8302, -79.5495) radius 1.6 construction
  circle A63 centre (37.8302, -79.5495) radius 1.6 construction
  circle A64 centre (20.5578, -60.8546) radius 1.55 construction
  circle A65 centre (-20.5578, -60.8546) radius 1.55 construction
  circle A66 centre (79.5495, 37.8302) radius 1.6 construction
  circle A67 centre (37.8302, 79.5495) radius 1.6 construction
  circle A68 centre (79.5495, -37.8302) radius 1.6 construction
  circle A69 centre (-79.5495, -37.8302) radius 1.6 construction
  circle A70 centre (-79.5495, 37.8302) radius 1.6 construction
  circle A71 centre (-37.8302, 79.5495) radius 1.6 construction
  circle A72 centre (22, 0) radius 1.6 construction
  circle A73 centre (0, -22) radius 1.6 construction
  circle A74 centre (-22, 0) radius 1.6 construction
  circle A75 centre (0, 22) radius 1.6 construction
  circle A76 centre (43.1335, -21.9203) radius 1.6 construction
  circle A77 centre (0, 0) radius 18 construction
  circle A78 centre (-43.1335, 21.9203) radius 1.6 construction
  circle A79 centre (-21.9203, -43.1335) radius 1.6 construction
  circle A80 centre (21.9203, 43.1335) radius 1.6 construction
  circle A81 centre (43.1335, 21.9203) radius 1.6 construction
  circle A82 centre (-43.1335, -21.9203) radius 1.6 construction
  line L53 (-23.6881, -37.8302) -> (-37.8302, -23.6881) projected
  arc A83 (-37.8302, -20.8597) -> (-37.8302, -23.6881) centre (-36.416, -22.2739) ccw construction
  line L54 (-37.8302, -20.8597) -> (-24.6871, -7.7166) construction
  arc A84 (-21.4111, -8.4003) -> (-24.6871, -7.7166) centre (-23.2729, -9.1308) ccw construction
  arc A85 (-21.4111, -8.4003) -> (-8.4003, -21.4111) centre (0, 0) ccw construction
  arc A86 (-7.7166, -24.6871) -> (-8.4003, -21.4111) centre (-9.1308, -23.2729) ccw construction
  line L55 (-7.7166, -24.6871) -> (-20.8597, -37.8302) projected
  arc A87 (-23.6881, -37.8302) -> (-20.8597, -37.8302) centre (-22.2739, -36.416) ccw projected
  circle A88 centre (21.9203, -43.1335) radius 1.6 construction
  line L56 (37.8302, 20.8597) -> (24.6871, 7.7166) construction
  arc A89 (21.4111, 8.4003) -> (24.6871, 7.7166) centre (23.2729, 9.1308) ccw construction
  arc A90 (21.4111, 8.4003) -> (8.4003, 21.4111) centre (0, 0) ccw construction
  arc A91 (7.7166, 24.6871) -> (8.4003, 21.4111) centre (9.1308, 23.2729) ccw construction
  line L57 (7.7166, 24.6871) -> (20.8597, 37.8302) construction
  arc A92 (23.6881, 37.8302) -> (20.8597, 37.8302) centre (22.2739, 36.416) ccw construction
  line L58 (23.6881, 37.8302) -> (37.8302, 23.6881) construction
  arc A93 (37.8302, 20.8597) -> (37.8302, 23.6881) centre (36.416, 22.2739) ccw construction
  arc A94 (-24.6871, 7.7166) -> (-21.4111, 8.4003) centre (-23.2729, 9.1308) ccw construction
  line L59 (-24.6871, 7.7166) -> (-37.8302, 20.8597) construction
  arc A95 (-37.8302, 23.6881) -> (-37.8302, 20.8597) centre (-36.416, 22.2739) ccw construction
  line L60 (-37.8302, 23.6881) -> (-23.6881, 37.8302) construction
  arc A96 (-20.8597, 37.8302) -> (-23.6881, 37.8302) centre (-22.2739, 36.416) ccw construction
  line L61 (-20.8597, 37.8302) -> (-7.7166, 24.6871) construction
  arc A97 (-8.4003, 21.4111) -> (-7.7166, 24.6871) centre (-9.1308, 23.2729) ccw construction
  arc A98 (-8.4003, 21.4111) -> (-21.4111, 8.4003) centre (0, 0) ccw construction
  circle A99 centre (-21.9203, 43.1335) radius 1.6 construction
  arc A100 (8.4003, -21.4111) -> (7.7166, -24.6871) centre (9.1308, -23.2729) ccw construction
  arc A101 (8.4003, -21.4111) -> (21.4111, -8.4003) centre (0, 0) ccw construction
  arc A102 (24.6871, -7.7166) -> (21.4111, -8.4003) centre (23.2729, -9.1308) ccw construction
  line L62 (24.6871, -7.7166) -> (37.8302, -20.8597) construction
  arc A103 (37.8302, -23.6881) -> (37.8302, -20.8597) centre (36.416, -22.2739) ccw construction
  line L63 (37.8302, -23.6881) -> (23.6881, -37.8302) projected
  arc A104 (20.8597, -37.8302) -> (23.6881, -37.8302) centre (22.2739, -36.416) ccw projected
  line L64 (20.8597, -37.8302) -> (7.7166, -24.6871) projected
  line L65 (-46.669, 63.6396) -> (-27.2236, 44.1942) construction
  arc A105 (-27.2236, 41.3657) -> (-27.2236, 44.1942) centre (-28.6378, 42.78) ccw construction
  line L66 (-27.2236, 41.3657) -> (-41.3657, 27.2236) construction
  arc A106 (-44.1942, 27.2236) -> (-41.3657, 27.2236) centre (-42.78, 28.6378) ccw construction
  line L67 (-44.1942, 27.2236) -> (-63.6396, 46.669) construction
  line L68 (-63.6396, 46.669) -> (-46.669, 63.6396) construction
  line L69 (63.6396, 46.669) -> (44.1942, 27.2236) construction
  arc A107 (41.3657, 27.2236) -> (44.1942, 27.2236) centre (42.78, 28.6378) ccw construction
  line L70 (41.3657, 27.2236) -> (27.2236, 41.3657) construction
  arc A108 (27.2236, 44.1942) -> (27.2236, 41.3657) centre (28.6378, 42.78) ccw construction
  line L71 (27.2236, 44.1942) -> (46.669, 63.6396) construction
  line L72 (46.669, 63.6396) -> (63.6396, 46.669) construction
  line L73 (46.669, -63.6396) -> (27.2236, -44.1942) construction
  arc A109 (27.2236, -41.3657) -> (27.2236, -44.1942) centre (28.6378, -42.78) ccw construction
  line L74 (27.2236, -41.3657) -> (41.3657, -27.2236) construction
  arc A110 (44.1942, -27.2236) -> (41.3657, -27.2236) centre (42.78, -28.6378) ccw construction
  line L75 (44.1942, -27.2236) -> (63.6396, -46.669) construction
  line L76 (63.6396, -46.669) -> (46.669, -63.6396) construction
  arc A111 (3.4868, -52.0398) -> (5.1776, -53.4237) centre (6.1018, -50.5696) ccw construction
  arc A112 (3.4868, -52.0398) -> (-3.4868, -52.0398) centre (0, -54) ccw construction
  arc A113 (-5.1776, -53.4237) -> (-3.4868, -52.0398) centre (-6.1018, -50.5696) ccw construction
  line L77 (-5.1776, -53.4237) -> (-14.5119, -56.4463) construction
  arc A114 (-15.1585, -56.5907) -> (-14.5119, -56.4463) centre (-15.6055, -53.069) ccw construction
  line L78 (-15.1585, -56.5907) -> (-20.596, -57.2809) construction
  line L79 (-20.596, -57.2809) -> (-26.2105, -51.6664) construction
  line L80 (-26.2105, -51.6664) -> (-21.6698, -47.1257) construction
  arc A115 (-21.6698, -47.1257) -> (-17.9282, -43.384) centre (-21.9203, -43.1335) ccw construction
  line L81 (-17.9282, -43.384) -> (-1.4142, -26.8701) construction
  arc A116 (1.4142, -26.8701) -> (-1.4142, -26.8701) centre (0, -28.2843) ccw construction
  line L82 (1.4142, -26.8701) -> (17.9282, -43.384) construction
  arc A117 (17.9282, -43.384) -> (21.6698, -47.1257) centre (21.9203, -43.1335) ccw construction
  line L83 (21.6698, -47.1257) -> (26.2105, -51.6664) construction
  line L84 (26.2105, -51.6664) -> (20.596, -57.2809) construction
  line L85 (20.596, -57.2809) -> (15.1585, -56.5907) construction
  arc A118 (14.5119, -56.4463) -> (15.1585, -56.5907) centre (15.6055, -53.069) ccw construction
  line L86 (14.5119, -56.4463) -> (5.1776, -53.4237) construction
  arc A119 (90.4395, -37.7453) -> (97.9653, -2.6059) centre (0, 0) ccw construction
  arc A120 (87.1795, -38.3892) -> (90.4395, -37.7453) centre (88.5938, -36.975) ccw construction
  line L87 (87.1795, -38.3892) -> (83.085, -34.2947) construction
  arc A121 (83.085, -34.2947) -> (76.014, -34.2947) centre (79.5495, -37.8302) ccw construction
  line L88 (76.014, -34.2947) -> (67.8823, -42.4264) construction
  line L89 (67.8823, -42.4264) -> (47.1257, -21.6698) construction
  arc A122 (47.1257, -21.6698) -> (43.384, -17.9282) centre (43.1335, -21.9203) ccw construction
  line L90 (43.384, -17.9282) -> (26.8701, -1.4142) construction
  arc A123 (26.8701, 1.4142) -> (26.8701, -1.4142) centre (28.2843, 0) ccw construction
  line L91 (26.8701, 1.4142) -> (43.384, 17.9282) construction
  arc A124 (43.384, 17.9282) -> (47.1257, 21.6698) centre (43.1335, 21.9203) ccw construction
  line L92 (47.1257, 21.6698) -> (67.8823, 42.4264) construction
  line L93 (67.8823, 42.4264) -> (76.014, 34.2947) construction
  arc A125 (76.014, 34.2947) -> (83.085, 34.2947) centre (79.5495, 37.8302) ccw construction
  line L94 (83.085, 34.2947) -> (87.1795, 38.3892) construction
  arc A126 (90.4395, 37.7453) -> (87.1795, 38.3892) centre (88.5938, 36.975) ccw construction
  arc A127 (97.9653, 2.6059) -> (90.4395, 37.7453) centre (0, 0) ccw construction
  arc A128 (97.9653, 2.6059) -> (97.9653, -2.6059) centre (101, 0) ccw construction
  circle A129 centre (-101, 0) radius 1.6 construction
  circle A130 centre (101, 0) radius 1.6 construction
  circle A131 centre (90.3659, 45.1111) radius 1.6 construction
  circle A132 centre (-90.3659, -45.1111) radius 1.6 construction
  circle A133 centre (45.1111, 90.3659) radius 1.6 construction
  circle A134 centre (-45.1111, -90.3659) radius 1.6 construction
  circle A135 centre (90.3659, -45.1111) radius 1.6 construction
  circle A136 centre (-90.3659, 45.1111) radius 1.6 construction
  circle A137 centre (-45.1111, 90.3659) radius 1.6 construction
  circle A138 centre (45.1111, -90.3659) radius 1.6 construction
  line L95 (-21.9203, -43.1335) -> (-21.9203, -26.8701) construction
  line L96 (-37.8302, -23.6881) -> (-23.6881, -37.8302) projected
  line L97 (-27.981, -33.5373) -> (-23.3345, -28.8909)
  line L98 (-27.981, -33.5373) -> (-21.4099, -33.5373) construction
  line L99 (-20.5061, -28.8909) -> (-16.2132, -33.1838)
  line L100 (-20.8597, -37.8302) -> (-7.7166, -24.6871) projected
  line L101 (-21.9203, -27.4767) -> (-15.8492, -27.4767) construction
  arc A139 (-20.5061, -28.8909) -> (-23.3345, -28.8909) centre (-21.9203, -30.3051) ccw
  line L102 (27.981, -33.5373) -> (23.3345, -28.8909)
  line L103 (20.5061, -28.8909) -> (16.2132, -33.1838)
  arc A140 (23.3345, -28.8909) -> (20.5061, -28.8909) centre (21.9203, -30.3051) ccw
  circle A141 centre (21.9203, -33.1335) radius 1.6
  circle A142 centre (31.9203, -33.1335) radius 1.6
  line L104 (43.1335, -21.9203) -> (21.9203, -43.1335) construction
  line L105 (-21.9203, -33.1335) -> (21.9203, -33.1335) construction
  arc A143 (27.9446, -33.5737) -> (32.3605, -29.1578) centre (31.9203, -33.1335) ccw
  line L106 (37.8302, -23.6881) -> (23.6881, -37.8302) construction
  arc A144 (27.9365, -33.4928) -> (27.9446, -33.5737) centre (31.9203, -33.1335) ccw
  arc A145 (32.3605, -29.1578) -> (27.9365, -33.4928) centre (31.9203, -33.1335) ccw construction
  circle A146 centre (-31.9203, -33.1335) radius 1.6
  arc A147 (-32.3605, -29.1578) -> (-27.9446, -33.5737) centre (-31.9203, -33.1335) ccw
  line L107 (21.9203, -28.3051) -> (33.2132, -28.3051)
  line L108 (-21.9203, -28.3051) -> (-33.2132, -28.3051)
  point P0 (23.5772, -29.1335)
  dimension "d127" = 3.2
  dimension "d128" = 10
  dimension "d129" = 45
  dimension "d130" = 45
  dimension "d131" = 4
  dimension "d132" = 4
  dimension "d133" = 2
  dimension "d136" = 3.2
  dimension "d137" = 31.9203
  dimension "d138" = 8
  constraints: 24 end point, 13 point on circle, 12 point on line, 12 symmetric about line, 10 centre point, 4 horizontal, 3 tangent, 3 vertical, 2 coincident, 2 equal length, 4 other
  measures "d127" diameter of A0
  measures "d128" distance of A79.centre L105.start
  measures "d129" angle of L98 L97
  measures "d130" angle of L99 L101
  measures "d131" distance from line of L105.start L99
  measures "d132" distance from line of L97 L105.start
  measures "d133" radius of A139
  measures "d136" diameter of A142
  measures "d137" distance from line of L0 A142.centre
  measures "d138" diameter of A143
extrude "Выдавливание11" add sketch "Эскиз9" against normal up to surface (2 mm away)
extrude "Выдавливание12" cut sketch "Эскиз9" along normal mid plane 33.2 contours A142 | A146